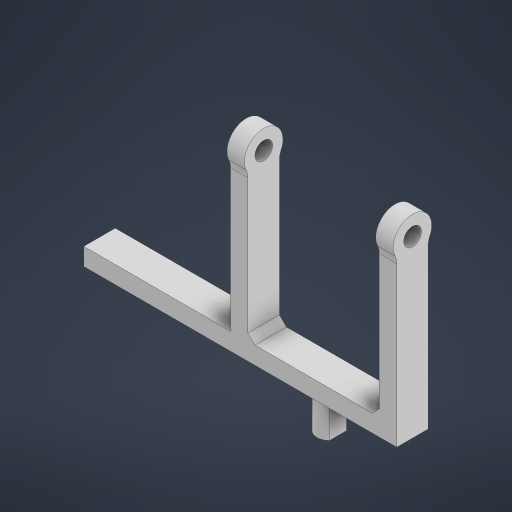
# Autodesk Inventor part: gunholder_clip
Saved by Autodesk Inventor 2024 (Build 280153000, 153)
## iProperties
Created: 2023-06-15
Part Number: gunholder_clip
Material: 일반
Document SubType Name: Modeling
Designer: 6gioc
Density: 1 g/cm^3
Appearance: 기본값
Author: 6gioc
Autodesk Inventor part; units mm, degrees
ref_plane "YZ Plane" through (0, 0, 0) normal (1, 0, 0) x (0, 1, 0)
ref_plane "XZ Plane" through (0, 0, 0) normal (0, 1, 0) x (-1, 0, 0)
ref_plane "XY Plane" through (0, 0, 0) normal (0, 0, 1) x (1, 0, 0)
sketch "스케치4" plane through (0, 0, 0) normal (1, 0, 0) x (0, 1, 0)
  circle A0 centre (0, 0) radius 2.5
  circle A1 centre (0, 0) radius 5.5
  circle A2 centre (0, 0) radius 4.5
  line L0 (0, -4.5) -> (-50, -4.5)
  line L1 (-50, -4.5) -> (-50, 4.5)
  line L2 (-50, 4.5) -> (0, 4.5)
  line L3 (0, 4.5) -> (0, -4.5)
  point P0 (-3.1623, -4.5)
  point P1 (-3.1623, 4.5)
  dimension "d17" = 9
  dimension "d15" = 5
  dimension "d16" = 11
  dimension "d18" = 50
  dimension "d19" = 9
  constraints: 8 end point, 3 coincident, 2 centre point, 2 parallel, 1 horizontal, 1 perpendicular, 1 vertical alignment, 2 other
  measures "d15" diameter of A0
  measures "d16" diameter of A1
  measures "d18" distance of L1.end L2.end
  measures "d19" distance of L0.end L1.end
extrude "돌출4" add sketch "스케치4" along normal blind 5 contours A0 L3 A2 | A0 L3 A2 | L2 A1 L0 A2 | A2 L0 A1 L2 | A1 L0 L1 L2
sketch "스케치5" plane through (5, 0, 0) normal (1, 0, 0) x (0, 0, -1)
  line L0 (-4.5, -50) -> (4.5, -50) projected
  line L1 (-4.5, -50) -> (4.5, -50)
  line L2 (4.5, -50) -> (4.5, -45)
  line L3 (4.5, -45) -> (-4.5, -45)
  line L4 (-4.5, -45) -> (-4.5, -50)
  point P0 (0, 0)
  dimension "d22" = 9
  dimension "d23" = 5
  constraints: 8 end point, 2 parallel, 1 horizontal, 1 perpendicular
  measures "d22" distance of L3.end L2.end
  measures "d23" distance of L2.end L1.end
extrude "돌출5" add sketch "스케치5" along normal blind 37.6
sketch "스케치6" plane through (42.6, 0, 0) normal (1, 0, 0) x (0, 0, -1)
  line L0 (-4.5, -50) -> (4.5, -50)
  line L1 (4.5, -50) -> (4.5, 0)
  line L2 (4.5, 0) -> (-4.5, 0)
  line L3 (-4.5, 0) -> (-4.5, -50)
  circle A0 centre (0, 0) radius 4.5
  circle A1 centre (0, 0) radius 5.5
  circle A2 centre (0, 0) radius 2.5
  point P0 (-4.5, -3.1623)
  point P1 (4.5, -3.1623)
  dimension "d26" = 9
  dimension "d27" = 50
  dimension "d28" = 11
  dimension "d29" = 5
  constraints: 8 end point, 3 coincident, 2 centre point, 2 parallel, 1 horizontal, 1 horizontal alignment, 1 perpendicular, 2 other
  measures "d26" distance of L2.end L1.end
  measures "d27" distance of L1.end L0.end
  measures "d28" diameter of A1
  measures "d29" diameter of A2
extrude "돌출6" add sketch "스케치6" along normal blind 5 contours L3 A1 L1 L0 | A1 L1 A0 L3 | L3 A0 L1 A1 | A0 L2 A2 | L2 A2 A0
fillet "모깎기1" radius 5 4 edges at (45.1, -3.1623, 4.5) (2.5, -3.1623, 4.5) (45.1, -3.1623, -4.5) (2.5, -3.1623, -4.5)
chamfer "모따기1" distance 2 angle 45 2 edges at (5, -45, 0) (42.6, -45, 0)
sketch "스케치7" plane through (0, -50, -4.5) normal (0, -1, 0) x (1, 0, 0)
  line L0 (0, 0) -> (47.6, 0) projected
  line L1 (47.6, 9) -> (47.6, 0) projected
  line L2 (0, 9) -> (47.6, 9) projected
  line L3 (0, 9) -> (47.6, 0)
  line L4 (47.6, 9) -> (0, 0)
  circle A0 centre (23.8, 4.5) radius 3.5
  line L5 (23.8, 4.5) -> (27.3, 4.5)
  line L6 (26.3, 4.5) -> (26.3, 6.9495)
  line L7 (26.3, 4.5) -> (26.3, 2.0505)
  line L8 (23.8, 4.5) -> (20.3, 4.5)
  line L9 (21.3, 4.5) -> (21.3, 6.9495)
  line L10 (21.3, 4.5) -> (21.3, 2.0505)
  line L11 (21.3, 4.5) -> (21.3, 4.9727)
  line L12 (26.3, 4.5) -> (26.3, 4.9727)
  point P0 (0, 4.5)
  dimension "d39" = 7
  constraints: 20 end point, 8 point on line, 6 point on circle, 2 perpendicular, 1 centre point, 1 coincident, 1 horizontal, 1 midpoint
  measures "d39" diameter of A0
extrude "돌출7" add sketch "스케치7" along normal blind 10 contours L10 L8 L4 | L4 L3 L7 A0 L10 | L3 L5 L7 | L8 L9 L3 | L3 L9 A0 L6 L4 | L4 L6 L5
extrude "돌출8" add sketch "스케치7" along normal blind 2 contours A0 L8 L10 L4 | L4 L10 A0 | A0 L7 L3 | L3 L7 L5 A0 | A0 L3 L9 L8 | A0 L5 L6 L4 | L4 L6 A0 | A0 L9 L3
sketch "스케치8" plane through (0, 0, 0) normal (-1, 0, 0) x (0, 0, 1)
  line L0 (4.5, -50) -> (-4.5, -50) projected
  line L1 (-4.5, -50) -> (4.5, -50)
  line L2 (4.5, -50) -> (4.5, -45)
  line L3 (4.5, -45) -> (-4.5, -45)
  line L4 (-4.5, -45) -> (-4.5, -50)
  point P0 (0, 0)
  dimension "d45" = 9
  dimension "d46" = 5
  constraints: 8 end point, 2 parallel, 1 horizontal, 1 perpendicular
  measures "d45" distance of L3.end L2.end
  measures "d46" distance of L2.end L1.end
extrude "돌출9" add sketch "스케치8" along normal blind 42
